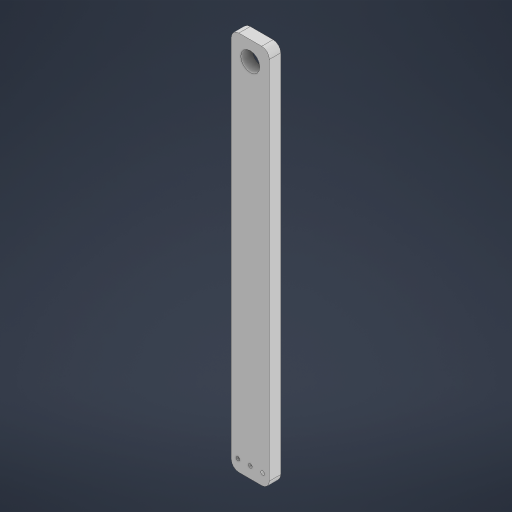
# Autodesk Inventor part: FP V2 Servo Arm v2
Saved by Autodesk Inventor 2023.6 (Build 276521000, 521)
## iProperties
Created: 2026-02-24
Part Number: FP V2 Servo Arm v2
Material: Generic
Document SubType Name: Modeling
Designer: user
Density: 1 g/cm^3
Appearance: Default
Author: user
Autodesk Inventor part; units mm, degrees
ref_plane "YZ Plane" through (0, 0, 0) normal (1, 0, 0) x (0, 1, 0)
ref_plane "XZ Plane" through (0, 0, 0) normal (0, 1, 0) x (-1, 0, 0)
ref_plane "XY Plane" through (0, 0, 0) normal (0, 0, 1) x (1, 0, 0)
sketch "Sketch1" plane through (0, 0, 0) normal (0, 0, 1) x (1, 0, 0)
  circle A0 centre (0, 0) radius 0.5
  line L0 (-3, 97) -> (3, 97)
  line L1 (5, 95) -> (5, -1)
  line L2 (3, -3) -> (-3, -3)
  line L3 (-5, -1) -> (-5, 95)
  arc A1 (-3, 97) -> (-5, 95) centre (-3, 95) ccw
  arc A2 (5, 95) -> (3, 97) centre (3, 95) ccw
  arc A3 (-5, -1) -> (-3, -3) centre (-3, -1) ccw
  arc A4 (3, -3) -> (5, -1) centre (3, -1) ccw
  circle A5 centre (0, 92) radius 2.5
  line L4 (0, 97) -> (0, 86.8445)
  circle A6 centre (-3.25, 0) radius 0.5
  circle A7 centre (3.25, 0) radius 0.5
  point P0 (-5, 97)
  point P1 (-5, -3)
  point P2 (0, -3)
  dimension "d3" = 1
  dimension "d7" = 100
  dimension "d8" = 10
  dimension "d9" = 3
  dimension "d10" = 2
  dimension "d11" = 5
  dimension "d12" = 5
  dimension "d15" = 1
  dimension "d16" = 1
  dimension "d17" = 3.25
  dimension "d18" = 3.25
  constraints: 10 end point, 8 centre point, 8 point on circle, 8 tangent, 5 point on line, 3 equal radius, 2 midpoint, 2 parallel, 1 horizontal, 1 perpendicular, 1 vertical
  measures "d3" diameter of A0
  measures "d7" distance of point (-5, -3) point (-5, 97)
  measures "d8" distance between parallel lines of L1 L3
  measures "d9" distance from line of L2 point (0, 0)
  measures "d10" radius of A1
  measures "d11" diameter of A5
  measures "d12" distance from line of L0 A5.centre
  measures "d15" diameter of A6
  measures "d16" diameter of A7
  measures "d17" distance of point (0, 0) A6.centre
  measures "d18" distance of A7.centre point (0, 0)
extrude "Extrusion1" add sketch "Sketch1" along normal blind 3
body "Solid1"
